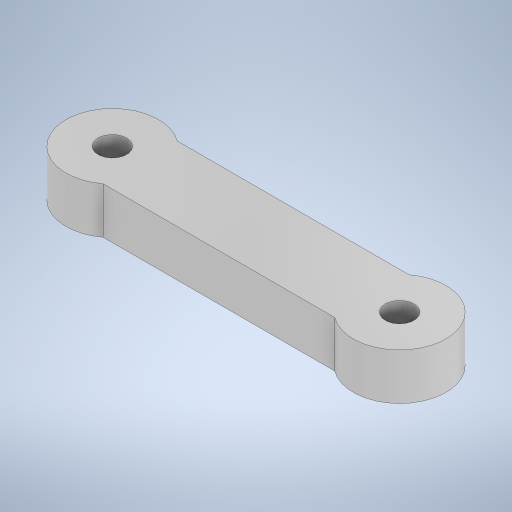
# Autodesk Inventor part: gripper_hand_connector
Saved by Autodesk Inventor 2024.2 (Build 282272000, 272)
## iProperties
Created: 2023-09-08
Part Number: gripper_hand_connector
Material: Aluminum 6061-AHC
Document SubType Name: Modeling
Designer: 박동준
Density: 2.7 g/cm^3
Appearance: Aluminum - Dark
Author: 박동준
Autodesk Inventor part; units mm, degrees
ref_plane "YZ Plane" through (0, 0, 0) normal (1, 0, 0) x (0, 1, 0)
ref_plane "XZ Plane" through (0, 0, 0) normal (0, 1, 0) x (-1, 0, 0)
sketch "Sketch1" plane through (0, 0, 0) normal (0, 1, 0) x (-1, 0, 0)
  circle A0 centre (0, 0) radius 5
  circle A1 centre (-31, 0) radius 5
  line L0 (-3, -4) -> (-28, -4)
  line L1 (-3, 4) -> (-28, 4)
  line L2 (0, 0) -> (-31, 0) construction
  dimension "d0" = 10
  dimension "d1" = 10
  dimension "d2" = 4
  dimension "d3" = 4
  dimension "d27" = 25
  constraints: 6 end point, 4 point on circle, 2 centre point, 2 parallel, 1 coincident, 1 horizontal
  measures "d0" diameter of A0
  measures "d1" diameter of A1
  measures "d2" distance between parallel lines of L0 L2
  measures "d3" distance between parallel lines of L1 L2
  measures "d27" distance of L0.start L0.end
extrude "Extrusion1" add sketch "Sketch1" along normal blind 5
sketch "Sketch2" plane through (0, 0, 0) normal (0, -1, 0) x (1, 0, 0)
  line L0 (0, 0) -> (31, 0) construction
  arc A0 (28, -4) -> (28, 4) centre (31, 0) ccw projected
  line L1 (3, 4) -> (28, 4) projected
  arc A1 (3, 4) -> (3, -4) centre (0, 0) ccw projected
  line L2 (28, -4) -> (3, -4) projected
  constraints: 2 coincident
hole "Hole1" at (31, 0, 0) at (0, 0, 0) direction (0, 1, 0) diameter 3.1 end through all
ref_plane "Work Plane1" through (0, 1.5, 0) normal (0, 1, 0) x (1, 0, 0)
body "Solid1"
